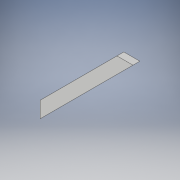
# Autodesk Inventor part: LBackAnglePiece
Saved by Autodesk Inventor 2018 (Build 220112000, 112)
## iProperties
Created: 2017-09-10
Part Number: LBackAnglePiece
Material: Generic
Document SubType Name: Modeling
Designer: jjsch
Density: 1 g/cm^3
Appearance: Default
Author: jjsch
Autodesk Inventor part; units mm, degrees
ref_plane "YZ Plane" through (0, 0, 0) normal (1, 0, 0) x (0, 1, 0)
ref_plane "XZ Plane" through (0, 0, 0) normal (0, 1, 0) x (-1, 0, 0)
ref_plane "XY Plane" through (0, 0, 0) normal (0, 0, 1) x (1, 0, 0)
sketch "Sketch1" plane through (0, 0, 0) normal (0, 0, 1) x (1, 0, 0)
  line L0 (514.35, 514.35) -> (0, 0)
  line L1 (0, 0) -> (0, 88.9)
  line L2 (0, 88.9) -> (425.45, 514.35)
  line L3 (425.45, 514.35) -> (514.35, 514.35)
  point P0 (514.35, 0)
  dimension "d0" = 88.9
  constraints: 8 end point, 1 coincident, 1 parallel, 1 perpendicular, 1 vertical
  measures "d0" distance of L0.end L1.end
extrude "Extrusion1" add sketch "Sketch1" along normal blind 38.1
body "Solid1"
